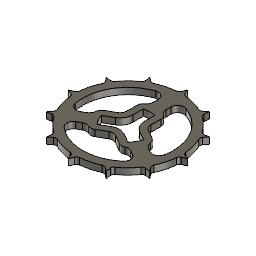
Small Cleat (Autodesk Fusion 360 design; units mm, degrees)
Autodesk Fusion 360 part; units mm, degrees
note: some values were not read from the file. Set by a fixed rule: which sketch regions a step uses.
sketch "Sketch2" plane through (0, 0, 0) normal (0, 0, 1) x (1, 0, 0)
  circle A0 centre (0, 0) radius 5 construction
  line L0 (0, 0) -> (0, 5) construction
  line L1 (0, 0) -> (4.3301, -2.5) construction
  line L2 (0, 0) -> (-4.3301, -2.5) construction
  line L3 (0, 0) -> (5, 0) construction
  circle A1 centre (-4.3301, -2.5) radius 1 construction
  circle A2 centre (4.3301, -2.5) radius 1 construction
  circle A3 centre (0, 5) radius 1 construction
  circle A4 centre (-4.3301, -2.5) radius 1.75
  circle A5 centre (4.3301, -2.5) radius 1.75
  circle A6 centre (0, 5) radius 1.75 construction
  circle A7 centre (0, 0) radius 6.75
  line L4 (4.3301, -2.5) -> (5.2051, -0.9845)
  line L5 (4.3301, -2.5) -> (3.4551, -4.0155)
  line L6 (0, 5) -> (1.75, 5)
  line L7 (0, 5) -> (-1.75, 5)
  line L8 (-4.3301, -2.5) -> (-3.4551, -4.0155)
  line L9 (-4.3301, -2.5) -> (-5.2051, -0.9845)
  circle A8 centre (0, 0) radius 2 construction
  line L10 (3.4551, -4.0155) -> (-0.0365, -1.9997)
  line L11 (5.2051, -0.9845) -> (1.7135, 1.0314)
  line L12 (1.75, 5) -> (1.75, 0.9682)
  line L13 (-1.75, 5) -> (-1.75, 0.9682)
  line L14 (-5.2051, -0.9845) -> (-1.7135, 1.0314)
  line L15 (-3.4551, -4.0155) -> (0.0365, -1.9997)
  line L16 (1.75, 5) -> (1.75, 6.5192)
  line L17 (-1.75, 5) -> (-1.75, 6.5192)
  line L18 (-3.4551, -4.0155) -> (-4.7708, -4.7751)
  line L19 (-5.2051, -0.9845) -> (-6.5208, -1.7441)
  line L20 (3.4551, -4.0155) -> (4.7708, -4.7751)
  line L21 (5.2051, -0.9845) -> (6.5208, -1.7441)
  circle A9 centre (0, 0) radius 8.75
  arc A10 (1.75, 3.3198) -> (3.75, -0.1443) centre (5.75, 3.3198) ccw
  arc A11 (-3.75, -0.1443) -> (-1.75, 3.3198) centre (-5.75, 3.3198) ccw
  arc A12 (2, -3.1754) -> (-2, -3.1754) centre (0, -6.6395) ccw
  circle A13 centre (-5.75, 3.3198) radius 2
  circle A14 centre (5.75, 3.3198) radius 2
  circle A15 centre (0, -6.6395) radius 2
  line L22 (0, -6.6395) -> (1, -4.9075)
  line L23 (0, -6.6395) -> (2, -6.6395) construction
  line L24 (0, -6.6395) -> (-1, -4.9075)
  line L25 (-1, -4.9075) -> (-4.9715, -7.2004)
  line L26 (1, -4.9075) -> (4.9715, -7.2004)
  line L27 (5.75, 3.3198) -> (4.75, 1.5877)
  line L28 (4.75, 1.5877) -> (8.7215, -0.7053)
  line L29 (5.75, 3.3198) -> (3.75, 3.3198)
  line L30 (3.75, 3.3198) -> (3.75, 7.9057)
  line L31 (-5.75, 3.3198) -> (-3.75, 3.3198)
  line L32 (-5.75, 3.3198) -> (-4.75, 1.5877)
  line L33 (-3.75, 3.3198) -> (-3.75, 7.9057)
  line L34 (-4.75, 1.5877) -> (-8.7215, -0.7053)
  circle A16 centre (-1.75, 6.5192) radius 2
  circle A17 centre (1.75, 6.5192) radius 2
  circle A18 centre (-6.5208, -1.7441) radius 2
  circle A19 centre (-4.7708, -4.7751) radius 2
  circle A20 centre (4.7708, -4.7751) radius 2
  circle A21 centre (6.5208, -1.7441) radius 2
  line L35 (4.3301, -2.5) -> (7.5777, -4.375)
  circle A22 centre (0, 0) radius 16.55
  circle A23 centre (0, 0) radius 16.55
  line L36 (4.7708, -4.7751) -> (4.6458, -4.9917)
  line L37 (6.5208, -1.7441) -> (6.6458, -1.5276)
  line L38 (-4.7708, -4.7751) -> (-4.6458, -4.9917)
  line L39 (-6.5208, -1.7441) -> (-6.6458, -1.5276)
  line L40 (1.75, 6.5192) -> (2, 6.5192)
  line L41 (-1.75, 6.5192) -> (-2, 6.5192)
  circle A24 centre (0, 0) radius 14.55
  line L42 (-2, 6.5192) -> (-2, 14.4119)
  line L43 (2, 6.5192) -> (2, 14.4119)
  line L44 (-6.6458, -1.5276) -> (-13.4811, -5.4739)
  line L45 (-4.6458, -4.9917) -> (-11.4811, -8.938)
  line L46 (4.6458, -4.9917) -> (11.4811, -8.938)
  line L47 (6.6458, -1.5276) -> (13.4811, -5.4739)
  line L48 (0, 0) -> (0, 16.55)
  line L49 (0, 16.55) -> (0, 18.55)
  line L50 (0, 18.55) -> (0.8372, 16.5288)
  line L51 (0, 18.55) -> (2.1877, 18.55) construction
  line L52 (0, 18.55) -> (-0.8372, 16.5288)
  line L53 (0, 18.55) -> (2.1877, 18.55) construction
  line L54 (-9.275, 16.0648) -> (-7.5394, 14.733)
  line L55 (-9.275, 16.0648) -> (-8.9894, 13.8958)
  line L56 (-16.0648, 9.275) -> (-13.8958, 8.9894)
  line L57 (-16.0648, 9.275) -> (-14.733, 7.5394)
  line L58 (-18.55, 0) -> (-16.5288, 0.8372)
  line L59 (-18.55, 0) -> (-16.5288, -0.8372)
  line L60 (-16.0648, -9.275) -> (-14.733, -7.5394)
  line L61 (-16.0648, -9.275) -> (-13.8958, -8.9894)
  line L62 (-9.275, -16.0648) -> (-8.9894, -13.8958)
  line L63 (-9.275, -16.0648) -> (-7.5394, -14.733)
  line L64 (0, -18.55) -> (-0.8372, -16.5288)
  line L65 (0, -18.55) -> (0.8372, -16.5288)
  line L66 (9.275, -16.0648) -> (7.5394, -14.733)
  line L67 (9.275, -16.0648) -> (8.9894, -13.8958)
  line L68 (16.0648, -9.275) -> (13.8958, -8.9894)
  line L69 (16.0648, -9.275) -> (14.733, -7.5394)
  line L70 (18.55, 0) -> (16.5288, -0.8372)
  line L71 (18.55, 0) -> (16.5288, 0.8372)
  line L72 (16.0648, 9.275) -> (14.733, 7.5394)
  line L73 (16.0648, 9.275) -> (13.8958, 8.9894)
  line L74 (9.275, 16.0648) -> (8.9894, 13.8958)
  line L75 (9.275, 16.0648) -> (7.5394, 14.733)
  circle A25 centre (0, 0) radius 14.05
  dimension "d35" = 10
  dimension "d36" = 60
  dimension "d37" = 150
  dimension "d38" = 2
  dimension "d39" = 2
  dimension "d40" = 2
  dimension "d41" = 3.5
  dimension "d42" = 3.5
  dimension "d43" = 3.5
  dimension "d44" = 4
  dimension "d46" = 4
  dimension "d47" = 4
  dimension "d50" = 17.5
  dimension "d53" = 4
  dimension "d54" = 4
  dimension "d55" = 4
  dimension "d56" = 60
  dimension "d57" = 120
  dimension "d58" = 90
  dimension "d59" = 120
  dimension "d64" = 33.1
  dimension "d69" = 0.25
  dimension "d70" = 0.25
  dimension "d71" = 0.25
  dimension "d72" = 0.25
  dimension "d73" = 0.25
  dimension "d74" = 0.25
  dimension "d75" = 29.1
  dimension "d78" = 2
  dimension "d79" = 67.5
  dimension "d80" = 112.5
  dimension "d82" = 360
  dimension "d87" = 28.1
  constraint coincident A0.centre L0.start
  constraint coincident A0 L0.end
  constraint vertical L0
  constraint coincident A0 L1.end
  constraint horizontal L3
  constraint coincident A0 L2.end
  constraint coincident L2.end A1.centre
  constraint coincident L1.end A2.centre
  constraint coincident L0.end A3.centre
  constraint concentric A1 A4
  constraint concentric A2 A5
  constraint concentric A3 A6
  constraint tangent A4 A7
  constraint coincident A5 L4.end
  constraint tangent A0 L4
  constraint perpendicular L1 L4
  constraint coincident A5 L5.end
  constraint tangent A0 L5
  constraint coincident A6 L6.end
  constraint tangent A0 L6
  constraint horizontal L6
  constraint coincident A6 L7.end
  constraint tangent A0 L7
  constraint coincident A4 L8.end
  constraint tangent A0 L8
  constraint coincident A4 L9.end
  constraint tangent A0 L9
  constraint parallel L8 L9
  constraint coincident A8 L10.end
  constraint tangent A5 L10
  constraint coincident A8 L11.end
  constraint tangent A5 L11
  constraint coincident A8 L12.end
  constraint tangent A6 L12
  constraint coincident A8 L13.end
  constraint tangent A6 L13
  constraint coincident A8 L14.end
  constraint perpendicular L9 L14
  constraint coincident A8 L15.end
  constraint tangent A4 L15
  constraint tangent L10 A12
  constraint tangent L15 A12
  constraint tangent L11 A10
  constraint tangent L12 A10
  constraint tangent L13 A11
  constraint tangent L14 A11
  constraint coincident A7 L16.end
  constraint tangent A6 L16
  constraint coincident A7 L17.end
  constraint tangent A6 L17
  constraint coincident A7 L18.end
  constraint tangent A4 L18
  constraint coincident A7 L19.end
  constraint tangent A4 L19
  constraint coincident A7 L20.end
  constraint tangent A5 L20
  constraint coincident A7 L21.end
  constraint perpendicular L4 L21
  constraint concentric A7 A9
  constraint coincident L12 A10.start
  constraint coincident L11 A10.end
  constraint coincident L13 A11.end
  constraint coincident L14 A11.start
  constraint coincident L15 A12.end
  constraint coincident L10 A12.start
  constraint concentric A11 A13
  constraint concentric A10 A14
  constraint concentric A12 A15
  constraint horizontal L23
  constraint coincident A12.centre A15.centre
  constraint coincident A15 L22.end
  constraint coincident A15 L24.end
  constraint coincident A9 L25.end
  constraint tangent A15 L25
  constraint coincident A9 L26.end
  constraint tangent A15 L26
  constraint coincident A10.centre A14.centre
  constraint coincident A14 L27.end
  constraint coincident A9 L28.end
  constraint tangent A14 L28
  constraint horizontal L29
  constraint coincident A14 L29.end
  constraint coincident A9 L30.end
  constraint tangent A14 L30
  constraint horizontal L31
  constraint coincident A11.centre A13.centre
  constraint coincident A13 L31.end
  constraint coincident A13 L32.end
  constraint coincident A9 L33.end
  constraint tangent A13 L33
  constraint coincident A9 L34.end
  constraint tangent A13 L34
  constraint coincident L17.end A16.centre
  constraint tangent L33 A16
  constraint coincident L16.end A17.centre
  constraint tangent L30 A17
  constraint coincident L19.end A18.centre
  constraint tangent L34 A18
  constraint coincident L18.end A19.centre
  constraint tangent L25 A19
  constraint coincident L20.end A20.centre
  constraint tangent L26 A20
  constraint coincident L21.end A21.centre
  constraint tangent L28 A21
  constraint coincident A9 L35.end
  constraint perpendicular L5 L35
  constraint concentric A8 A22
  constraint concentric A9 A23
  constraint perpendicular L20 L36
  constraint perpendicular L21 L37
  constraint perpendicular L18 L38
  constraint perpendicular L19 L39
  constraint perpendicular L16 L40
  constraint perpendicular L17 L41
  constraint concentric A23 A24
  constraint coincident A24 L42.end
  constraint perpendicular L41 L42
  constraint coincident A24 L43.end
  constraint perpendicular L40 L43
  constraint coincident A24 L44.end
  constraint perpendicular L39 L44
  constraint coincident A24 L45.end
  constraint perpendicular L38 L45
  constraint coincident A24 L46.end
  constraint perpendicular L36 L46
  constraint coincident A24 L47.end
  constraint perpendicular L37 L47
  constraint coincident A23 L48.end
  constraint parallel L0 L48
  constraint parallel L48 L49
  constraint horizontal L51
  constraint coincident A22 L50.end
  constraint horizontal L53
  constraint coincident A23 L52.end
  measures "d35" diameter of A0
  measures "d36" angle of L0 L1
  measures "d37" angle of L2 L3
  measures "d38" diameter of A1
  measures "d39" diameter of A2
  measures "d40" diameter of A3
  measures "d41" diameter of A4
  measures "d42" diameter of A5
  measures "d43" diameter of A6
  measures "d44" diameter of A8
  measures "d46" radius of A10
  measures "d47" radius of A11
  measures "d50" diameter of A9
  measures "d53" diameter of A13
  measures "d54" diameter of A14
  measures "d55" diameter of A15
  measures "d56" angle of L22 L23
  measures "d57" angle of L22 L24
  measures "d58" angle of L26 L27
  measures "d59" angle of L31 L32
  measures "d64" diameter of A22
  measures "d69" distance of L20.end L36.end
  measures "d70" distance of L21.end L37.end
  measures "d71" distance of L18.end L38.end
  measures "d72" distance of L19.end L39.end
  measures "d73" distance of L16.end L40.end
  measures "d74" distance of L17.end L41.end
  measures "d75" diameter of A24
  measures "d78" distance of L48.end L49.end
  measures "d79" angle of L50 L51
  measures "d80" angle of L52 L53
  measures "d87" diameter of A25
extrude "Extrude4" add sketch "Sketch2" along normal blind 2 contours A7 L14 L19 A18 | A7 L13 L14 A11 A13 L33 L34 A16 A18 | A7 L15 L18 A19 | A7 L10 L15 A12 A15 L25 L26 A19 A20 | A7 A18 L39 L44 | A7 A18 A19 L39 L44 | A7 L34 A18 | A7 A18 A19 L38 L45 | A7 A19 L38 L45 | A7 A18 A19 | A7 L25 A19 | A9 A18 A19 L44 L45 | A7 L13 L17 A16 | A7 L10 L20 A20 | A9 L44 L45 A25 | A7 A16 L41 L42 | A7 L33 A16 | A7 L26 A20 | A7 A20 L36 L46 | A24 L44 L45 A25 | A24 L42 L44 A25 | A7 A16 A17 L41 L42 | A24 L45 L46 A25 | A7 A20 A21 L36 L46 | A9 L42 L48 A25 | A24 L42 L48 A25 | A7 A17 L48 | A7 A16 L48 | A9 A16 L42 L48 | A24 L46 L47 A25 | A9 L46 L47 A25 | A7 A21 L35 | A7 A20 L35 | A7 L11 L21 A21 | A7 L11 L12 A10 A14 L28 L30 A17 A21 | A9 L43 L48 A25 | A24 L43 L48 A25 | A7 A16 A17 L40 L43 | A9 A17 L43 L48 | A7 L12 L16 A17 | A9 A20 L35 L46 | A24 L43 L47 A25 | A7 A20 A21 L37 L47 | A9 A21 L35 L47 | A7 A21 L37 L47 | A7 L28 A21 | A7 A17 L40 L43 | A7 L30 A17 | A22 A23 | A22 A23 L70 L71 | A22 A23 L72 L73 | A22 A23 L68 L69 | A22 A23 L74 L75 | A22 A23 L66 L67 | A22 A23 L49 L50 | A22 A23 L64 L65 | A22 A23 L49 L52 | A22 A23 L62 L63 | A22 A23 L54 L55 | A22 A23 L60 L61 | A22 A23 L56 L57 | A22 A23 L58 L59 picked at (-0.1006, 7.0013) picked at (0.1006, 7.0013)
fillet "Fillet5" radius 2 12 edges at (-2, 13.9069, 1) (2, 13.9069, 1) (2, 8.5035, 1) (-2, 8.5035, 1) (-8.3643, -2.5197, 1) (-11.0437, -8.6855, 1) (-6.3643, -5.9838, 1) (-13.0437, -5.2214, 1) (6.3643, -5.9838, 1) (11.0437, -8.6855, 1) (13.0437, -5.2214, 1) (8.3643, -2.5197, 1)
fillet "Fillet6" radius 1 24 edges at (0.8372, 16.5288, 1) (8.9894, 13.8958, 1) (7.5394, 14.733, 1) (-7.5394, 14.733, 1) (-8.9894, 13.8958, 1) (-13.8958, 8.9894, 1) (-16.5288, 0.8372, 1) (-16.5288, -0.8372, 1) (-14.733, -7.5394, 1) (-13.8958, -8.9894, 1) (-8.9894, -13.8958, 1) (-7.5394, -14.733, 1) (-0.8372, -16.5288, 1) (0.8372, -16.5288, 1) (7.5394, -14.733, 1) (8.9894, -13.8958, 1) (13.8958, -8.9894, 1) (14.733, -7.5394, 1) (16.5288, -0.8372, 1) (16.5288, 0.8372, 1) (-0.8372, 16.5288, 1) (-14.733, 7.5394, 1) (14.733, 7.5394, 1) (13.8958, 8.9894, 1)
equation "inner_diameter = 33.1 mm"
equation "outer_diameter = 37.1 mm"
equation "d87 = inner_inner_diameter"
equation "inner_inner_diameter = 28.1 mm"
